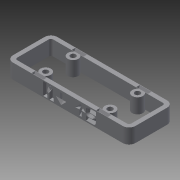
# Autodesk Inventor part: dualBaccable-ucan_fysect_middle
Saved by Autodesk Inventor 2014 SP2 (Build 180246200, 246)
## iProperties
Created: 2025-01-14
Part Number: dualBaccable-ucan_fysect_middle
Material: Generic
Document SubType Name: Sheet Metal
Designer: GauchoHP
Density: 1 g/cm^3
Sheet Metal Rule: Default_mm
Appearance: Default
Author: GauchoHP
Autodesk Inventor part; units mm, degrees
ref_plane "YZ Plane" through (0, 0, 0) normal (1, 0, 0) x (0, 1, 0)
ref_plane "XZ Plane" through (0, 0, 0) normal (0, 1, 0) x (-1, 0, 0)
ref_plane "XY Plane" through (0, 0, 0) normal (0, 0, 1) x (1, 0, 0)
sketch "Sketch1" plane through (0, 0, 0) normal (0, 0, 1) x (1, 0, 0)
  line L0 (-8.892067, 9.824871) -> (43.107933, 9.824871)
  line L1 (46.107933, 6.824871) -> (46.107933, -8.175129)
  line L2 (43.107933, -11.175129) -> (-8.892067, -11.175129)
  line L3 (-11.892067, -8.175129) -> (-11.892067, 6.824871)
  arc A0 (-8.892067, 9.824871) -> (-11.892067, 6.824871) centre (-8.892067, 6.824871) ccw
  arc A1 (46.107933, 6.824871) -> (43.107933, 9.824871) centre (43.107933, 6.824871) ccw
  arc A2 (43.107933, -11.175129) -> (46.107933, -8.175129) centre (43.107933, -8.175129) ccw
  arc A3 (-11.892067, -8.175129) -> (-8.892067, -11.175129) centre (-8.892067, -8.175129) ccw
  line L4 (43.107933, 7.824871) -> (-8.892067, 7.824871)
  arc A4 (-8.892067, 7.824871) -> (-9.892067, 6.824871) centre (-8.892067, 6.824871) ccw
  line L5 (-9.892067, 6.824871) -> (-9.892067, -8.175129)
  arc A5 (-9.892067, -8.175129) -> (-8.892067, -9.175129) centre (-8.892067, -8.175129) ccw
  line L6 (-8.892067, -9.175129) -> (43.107933, -9.175129)
  arc A6 (43.107933, -9.175129) -> (44.107933, -8.175129) centre (43.107933, -8.175129) ccw
  line L7 (44.107933, -8.175129) -> (44.107933, 6.824871)
  arc A7 (44.107933, 6.824871) -> (43.107933, 7.824871) centre (43.107933, 6.824871) ccw
  circle A8 centre (2.607933, -7.175129) radius 2.5
  circle A9 centre (2.607933, -7.175129) radius 1.25
  circle A10 centre (2.607933, 5.824871) radius 2.5
  circle A11 centre (2.607933, 5.824871) radius 1.25
  circle A12 centre (33.107933, 5.824871) radius 2.5
  circle A13 centre (33.107933, 5.824871) radius 1.25
  circle A14 centre (33.107933, -7.175129) radius 2.5
  circle A15 centre (33.107933, -7.175129) radius 1.25
  point P0 (0, 0)
  point P1 (-11.892067, 9.824871)
  point P2 (46.107933, 9.824871)
  point P3 (-11.892067, -11.175129)
  dimension "d0" = 58
  dimension "d1" = 21
  dimension "d2" = 3
  dimension "d5" = 2
  dimension "d6" = 5
  dimension "d7" = 2.5
  dimension "d8" = 5
  dimension "d9" = 2.5
  dimension "d10" = 5
  dimension "d11" = 2.5
  dimension "d12" = 5
  dimension "d13" = 2.5
  dimension "d14" = 30.5
  dimension "d15" = 30.5
  dimension "d16" = 13
  dimension "d17" = 2
  dimension "d18" = 11
  dimension "d19" = 11
  constraints: 16 centre point, 16 end point, 16 point on circle, 8 tangent, 6 point on line, 4 coincident, 4 parallel, 3 equal radius, 2 perpendicular, 1 horizontal, 7 other
  measures "d0" distance of point (-11.892, 9.825) point (46.108, 9.825)
  measures "d1" distance of point (-11.892, -11.175) point (-11.892, 9.825)
  measures "d2" radius of A0
  measures "d5" distance between parallel lines of L4 L0
  measures "d6" diameter of A8
  measures "d7" diameter of A9
  measures "d8" diameter of A10
  measures "d9" diameter of A11
  measures "d10" diameter of A12
  measures "d11" diameter of A13
  measures "d12" diameter of A14
  measures "d13" diameter of A15
  measures "d14" distance of A12.centre A10.centre
  measures "d15" distance of A14.centre A8.centre
  measures "d16" distance of A8.centre A10.centre
  measures "d17" distance from line of L6 A8.centre
  measures "d18" distance from line of L7 A12.centre
  measures "d19" distance from line of L7 A14.centre
extrude "Extrusion1" add sketch "Sketch1" along normal blind 7 contours L0 A1 L1 A2 L2 A3 L3 A0 | A12 L4 | L4 A12 | A10 L4 | L4 A10 | A14 L6 | L6 A14 | A8 L6 | L6 A8
sketch "Sketch2" plane through (0, 0, 7) normal (0, 0, 1) x (1, 0, 0)
  circle A0 centre (2.607933, 5.824871) radius 1.25
  line L0 (43.107933, 9.824871) -> (-8.892067, 9.824871)
  line L1 (-8.892067, -11.175129) -> (43.107933, -11.175129)
  circle A1 centre (33.107933, -7.175129) radius 1.25
  circle A2 centre (33.107933, 5.824871) radius 1.25
  circle A3 centre (2.607933, -7.175129) radius 1.25
  line L2 (-0.142067, 9.174871) -> (5.357933, 9.174871)
  line L3 (5.357933, 9.174871) -> (5.357933, 8.474871)
  line L4 (5.357933, 8.474871) -> (-0.142067, 8.474871)
  line L5 (-0.142067, 8.474871) -> (-0.142067, 9.174871)
  line L6 (35.857933, 9.174871) -> (30.357933, 9.174871)
  line L7 (30.357933, 9.174871) -> (30.357933, 8.474871)
  line L8 (30.357933, 8.474871) -> (35.857933, 8.474871)
  line L9 (35.857933, 8.474871) -> (35.857933, 9.174871)
  line L10 (30.357933, -9.825129) -> (35.857933, -9.825129)
  line L11 (35.857933, -9.825129) -> (35.857933, -10.525129)
  line L12 (35.857933, -10.525129) -> (30.357933, -10.525129)
  line L13 (30.357933, -10.525129) -> (30.357933, -9.825129)
  line L14 (-0.142067, -9.825129) -> (5.357933, -9.825129)
  line L15 (5.357933, -9.825129) -> (5.357933, -10.525129)
  line L16 (5.357933, -10.525129) -> (-0.142067, -10.525129)
  line L17 (-0.142067, -10.525129) -> (-0.142067, -9.825129)
  point P0 (0, 0)
  dimension "d20" = 5.5
  dimension "d21" = 0.7
  dimension "d22" = 0.65
  dimension "d23" = 2.75
  dimension "d24" = 0.7
  dimension "d25" = 0.65
  dimension "d27" = 5.5
  dimension "d29" = 2.75
  dimension "d30" = 5.5
  dimension "d31" = 0.7
  dimension "d32" = 0.65
  dimension "d33" = 2.75
  dimension "d34" = 0.7
  dimension "d35" = 5.5
  dimension "d36" = 2.75
  dimension "d37" = 0.65
  constraints: 32 end point, 8 parallel, 4 horizontal, 4 perpendicular
  measures "d20" distance of L2.start L2.end
  measures "d21" distance of L2.end L3.end
  measures "d22" distance between parallel lines of L0 L2
  measures "d23" distance from line of L3 A0.centre
  measures "d24" distance of L6.end L7.end
  measures "d25" distance between parallel lines of L0 L6
  measures "d27" distance of L6.start L6.end
  measures "d29" distance from line of L7 A2.centre
  measures "d30" distance of L10.start L10.end
  measures "d31" distance of L10.end L11.end
  measures "d32" distance between parallel lines of L1 L12
  measures "d33" distance from line of L13 A1.centre
  measures "d34" distance of L14.end L15.end
  measures "d35" distance of L14.start L14.end
  measures "d36" distance from line of L17 A3.centre
  measures "d37" distance between parallel lines of L1 L16
extrude "Extrusion2" cut sketch "Sketch2" against normal blind 1.2 contours L2 L3 L4 L5 | L9 L8 L7 L6 | L10 L11 L12 L13 | L14 L15 L16 L17
chamfer "Chamfer1" distance 0.5 distance2 1.2 1 edges at (2.6079, -9.8251, 7) measured on face at (2.6079, -9.3251, 7)
chamfer "Chamfer2" distance 0.5 distance2 1.2 1 edges at (2.6079, -10.5251, 7) measured on face at (2.6079, -10.6251, 7)
chamfer "Chamfer3" distance 0.5 distance2 1.2 1 edges at (33.1079, -9.8251, 7) measured on face at (33.1079, -9.3251, 7)
chamfer "Chamfer4" distance 0.5 distance2 1.2 1 edges at (33.1079, -10.5251, 7) measured on face at (33.1079, -10.6251, 7)
chamfer "Chamfer5" distance 0.5 distance2 1.2 1 edges at (33.1079, 8.4749, 7) measured on face at (33.1079, 7.9749, 7)
chamfer "Chamfer6" distance 0.5 distance2 1.2 1 edges at (33.1079, 9.1749, 7) measured on face at (33.1079, 9.6749, 7)
chamfer "Chamfer7" distance 0.5 distance2 1.2 1 edges at (2.6079, 8.4749, 7) measured on face at (2.6079, 7.9749, 7)
chamfer "Chamfer8" distance 0.5 distance2 1.2 1 edges at (2.6079, 9.1749, 7) measured on face at (2.6079, 9.6749, 7)
sketch "Sketch3" plane through (0, 0, 0) normal (0, 0, -1) x (-1, 0, 0)
  circle A0 centre (-2.607933, -7.175129) radius 1.25
  line L0 (-43.107933, -11.175129) -> (8.892067, -11.175129)
  line L1 (8.892067, 9.824871) -> (-43.107933, 9.824871)
  circle A1 centre (-33.107933, 5.824871) radius 1.25
  circle A2 centre (-33.107933, -7.175129) radius 1.25
  circle A3 centre (-2.607933, 5.824871) radius 1.25
  line L2 (0.142067, -10.525129) -> (-5.357933, -10.525129)
  line L3 (-5.357933, -10.525129) -> (-5.357933, -9.825129)
  line L4 (-5.357933, -9.825129) -> (0.142067, -9.825129)
  line L5 (0.142067, -9.825129) -> (0.142067, -10.525129)
  line L6 (-35.857933, -10.525129) -> (-30.357933, -10.525129)
  line L7 (-30.357933, -10.525129) -> (-30.357933, -9.825129)
  line L8 (-30.357933, -9.825129) -> (-35.857933, -9.825129)
  line L9 (-35.857933, -9.825129) -> (-35.857933, -10.525129)
  line L10 (-30.357933, 8.474871) -> (-35.857933, 8.474871)
  line L11 (-35.857933, 8.474871) -> (-35.857933, 9.174871)
  line L12 (-35.857933, 9.174871) -> (-30.357933, 9.174871)
  line L13 (-30.357933, 9.174871) -> (-30.357933, 8.474871)
  line L14 (0.142067, 8.474871) -> (-5.357933, 8.474871)
  line L15 (-5.357933, 8.474871) -> (-5.357933, 9.174871)
  line L16 (-5.357933, 9.174871) -> (0.142067, 9.174871)
  line L17 (0.142067, 9.174871) -> (0.142067, 8.474871)
  point P0 (0, 0)
  point P1 (0, -1.350259)
  dimension "d64" = 5.5
  dimension "d65" = 0.7
  dimension "d66" = 0.65
  dimension "d67" = 2.75
  dimension "d68" = 0.7
  dimension "d69" = 0.65
  dimension "d70" = 5.5
  dimension "d71" = 2.75
  dimension "d72" = 5.5
  dimension "d73" = 0.7
  dimension "d74" = 0.65
  dimension "d75" = 2.75
  dimension "d76" = 0.7
  dimension "d77" = 5.5
  dimension "d78" = 2.75
  dimension "d79" = 0.65
  constraints: 36 end point, 8 parallel, 4 centre point, 4 perpendicular
  measures "d64" distance of L2.start L2.end
  measures "d65" distance of L2.end L3.end
  measures "d66" distance between parallel lines of L0 L2
  measures "d67" distance from line of L3 A0.centre
  measures "d68" distance of L6.end L7.end
  measures "d69" distance between parallel lines of L0 L6
  measures "d70" distance of L6.start L6.end
  measures "d71" distance from line of L7 A2.centre
  measures "d72" distance of L10.start L10.end
  measures "d73" distance of L10.end L11.end
  measures "d74" distance between parallel lines of L1 L12
  measures "d75" distance from line of L13 A1.centre
  measures "d76" distance of L14.end L15.end
  measures "d77" distance of L14.start L14.end
  measures "d78" distance from line of L17 A3.centre
  measures "d79" distance between parallel lines of L1 L16
extrude "Extrusion3" cut sketch "Sketch3" against normal blind 1.2 contours L2 L3 L4 L5 | L9 L8 L7 L6 | L10 L11 L12 L13 | L14 L15 L16 L17
chamfer "Chamfer9" distance 0.5 distance2 1.2 1 edges at (33.1079, 8.4749, 0) measured on face at (33.1079, 7.9749, 0)
chamfer "Chamfer10" distance 0.5 distance2 1.2 1 edges at (33.1079, 9.1749, 0) measured on face at (33.1079, 9.6749, 0)
chamfer "Chamfer11" distance 0.5 distance2 1.2 1 edges at (33.1079, -10.5251, 0) measured on face at (33.1079, -11.0251, 0)
chamfer "Chamfer12" distance 0.5 distance2 1.2 1 edges at (33.1079, -9.8251, 0) measured on face at (33.1079, -9.3251, 0)
chamfer "Chamfer13" distance 0.5 distance2 1.2 1 edges at (2.6079, 9.1749, 0) measured on face at (2.6079, 9.2749, 0)
chamfer "Chamfer14" distance 0.5 distance2 1.2 1 edges at (2.6079, 8.4749, 0) measured on face at (2.6079, 7.9749, 0)
chamfer "Chamfer15" distance 0.5 distance2 1.2 1 edges at (2.6079, -9.8251, 0) measured on face at (2.6079, -9.3251, 0)
chamfer "Chamfer16" distance 0.5 distance2 1.2 1 edges at (2.6079, -10.5251, 0) measured on face at (2.6079, -10.6251, 0)
sketch "Sketch4" plane through (-8.892067, -11.175129, 0) normal (0, -1, 0) x (1, 0, 0)
  line L0 (52, 0) -> (0, 0)
  line L1 (14.81046, 1) -> (15.81046, 1)
  line L2 (15.81046, 1) -> (15.81046, 4.585786)
  line L3 (15.81046, 6) -> (14.81046, 6)
  line L4 (14.81046, 6) -> (14.81046, 1)
  line L5 (17.81046, 6) -> (18.81046, 6)
  line L6 (18.81046, 6) -> (18.81046, 3)
  line L7 (18.81046, 1) -> (17.81046, 1)
  line L8 (17.81046, 1) -> (17.81046, 4.585786)
  line L9 (15.81046, 6) -> (16.81046, 5)
  line L10 (16.81046, 5) -> (17.81046, 6)
  line L11 (15.81046, 4.585786) -> (16.81046, 3.585786)
  line L12 (16.81046, 3.585786) -> (17.81046, 4.585786)
  line L13 (21.331649, 2.5) -> (22.831649, 1)
  line L14 (22.831649, 1) -> (24.331649, 2.5)
  line L15 (23.331649, 6) -> (22.331649, 6)
  line L16 (23.331649, 2.5) -> (23.331649, 6)
  line L17 (21.331649, 2.5) -> (22.331649, 2.5)
  line L18 (23.331649, 2.5) -> (24.331649, 2.5)
  line L19 (22.331649, 6) -> (22.331649, 2.5)
  line L20 (33.5, 4.5) -> (32, 6)
  line L21 (32, 6) -> (30.5, 4.5)
  line L22 (31.5, 1) -> (32.5, 1)
  line L23 (31.5, 4.5) -> (31.5, 1)
  line L24 (33.5, 4.5) -> (32.5, 4.5)
  line L25 (31.5, 4.5) -> (30.5, 4.5)
  line L26 (32.5, 1) -> (32.5, 4.5)
  line L27 (36.5, 4) -> (38, 4)
  line L28 (37.5, 3) -> (36, 3)
  line L29 (35, 2) -> (37.5, 2)
  line L30 (38, 1) -> (35, 1)
  line L31 (35, 1) -> (35, 2)
  line L32 (36, 6) -> (39, 6)
  line L33 (39, 6) -> (39, 5)
  line L34 (39, 5) -> (36.5, 5)
  line L35 (35, 4) -> (35, 5)
  line L36 (39, 2) -> (39, 3)
  line L37 (18.81046, 1) -> (18.81046, 3)
  arc A0 (36, 6) -> (35, 5) centre (36, 5) ccw
  arc A1 (39, 3) -> (38, 4) centre (38, 3) ccw
  arc A2 (38, 1) -> (39, 2) centre (38, 2) ccw
  arc A3 (35, 4) -> (36, 3) centre (36, 4) ccw
  arc A4 (36.5, 5) -> (36.5, 4) centre (36.5, 4.5) ccw
  arc A5 (37.5, 2) -> (37.5, 3) centre (37.5, 2.5) ccw
  point P0 (8.892067, 0)
  dimension "d106" = 1
  dimension "d107" = 3
  dimension "d108" = 5
  dimension "d109" = 1
  dimension "d110" = 1
  dimension "d111" = 1
  dimension "d112" = 1
  dimension "d116" = 5
  dimension "d118" = 1
  dimension "d121" = 1
  dimension "d122" = 5
  dimension "d123" = 5
  dimension "d125" = 4
  dimension "d134" = 1
  constraints: 74 end point, 12 point on circle, 11 perpendicular, 10 parallel, 8 tangent, 6 centre point, 5 horizontal, 3 equal radius
  measures "d106" distance of L7.end L7.start
  measures "d107" distance of L6.end L5.end
  measures "d108" distance of L1.end L3.start
  measures "d109" distance of L1.end L1.start
  measures "d110" distance between parallel lines of L9 L11
  measures "d111" distance between parallel lines of L12 L10
  measures "d112" distance of L15.end L15.start
  measures "d116" distance between parallel lines of L3 L1
  measures "d118" distance of L26.start L23.end
  measures "d121" distance between parallel lines of L0 L22
  measures "d122" distance from line of L15 L13.end
  measures "d123" distance from line of L22 L20.end
  measures "d125" distance between parallel lines of L6 L4
  measures "d134" distance between parallel lines of L0 L1
extrude "Extrusion4" cut sketch "Sketch4" against normal blind 1
chamfer "Chamfer18" distance 0.4 angle 45 16 edges at (28.6079, -11.1751, 6) (26.4008, -11.1751, 5.7071) (26.1079, -11.1751, 4.5) (26.4008, -11.1751, 3.2929) (27.8579, -11.1751, 3) (29.1079, -11.1751, 2.5) (27.3579, -11.1751, 2) (30.1079, -11.1751, 5.5) (28.8579, -11.1751, 5) (27.1079, -11.1751, 4.5) (28.3579, -11.1751, 4) (29.815, -11.1751, 3.7071) (30.1079, -11.1751, 2.5) (29.815, -11.1751, 1.2929) (27.6079, -11.1751, 1) (26.1079, -11.1751, 1.5)
chamfer "Chamfer19" distance 1 angle 45 4 edges at (22.1079, -11.1751, 4.5) (24.1079, -11.1751, 4.5) (12.9396, -11.1751, 2.5) (14.9396, -11.1751, 2.5)
chamfer "Chamfer22" distance 1 angle 45 10 edges at (23.1079, -10.1751, 1) (21.6079, -10.1752, 4.5) (22.3579, -10.1751, 5.25) (24.6079, -10.1752, 4.5) (23.8579, -10.1751, 5.25) (12.4396, -10.1752, 2.5) (13.1896, -10.1751, 1.75) (15.4396, -10.1752, 2.5) (14.6896, -10.1751, 1.75) (13.9396, -10.1751, 6)
chamfer "Chamfer23" distance 0.5 angle 45 15 edges at (28.6079, -10.1751, 6) (26.4008, -10.1751, 5.7071) (26.1079, -10.1751, 4.5) (26.4008, -10.1751, 3.2929) (27.8579, -10.1751, 3) (29.1079, -10.1751, 2.5) (27.3579, -10.1751, 2) (28.3579, -10.1751, 4) (29.815, -10.1751, 3.7071) (30.1079, -10.1751, 2.5) (29.815, -10.1751, 1.2929) (27.6079, -10.1751, 1) (27.2543, -10.1751, 4.1465) (27.2544, -10.1751, 4.8536) (28.8579, -10.1751, 5)
chamfer "Chamfer24" distance 0.5 angle 45 12 edges at (6.4184, -11.1751, 6) (7.4184, -11.1751, 5.5) (8.4184, -11.1751, 5.5) (9.4184, -11.1751, 6) (9.9184, -11.1751, 3.5) (5.9184, -11.1751, 3.5) (6.4184, -11.1751, 1) (9.4184, -11.1751, 1) (8.9184, -11.1751, 2.7929) (6.9184, -11.1751, 2.7929) (7.4184, -11.1751, 4.0858) (8.4184, -11.1751, 4.0858)
chamfer "Chamfer25" distance 0.5 angle 45 12 edges at (6.4184, -10.6751, 1) (6.9184, -10.6751, 2.7929) (9.9184, -10.6751, 3.5) (9.4184, -10.6751, 1) (5.9184, -10.6751, 3.5) (6.4184, -10.6751, 6) (7.4184, -10.6751, 5.5) (8.4184, -10.6751, 5.5) (9.4184, -10.6751, 6) (8.9184, -10.6751, 2.7929) (8.4184, -10.6751, 4.0858) (7.4184, -10.6751, 4.0858)
equation "\"BendRadius\" = Thickness"
equation "\"BendReliefWidth\" = Thickness"
equation "\"BendReliefDepth\" = 0.5 * Thickness"
equation "\"CornerReliefSize\" = 4 * Thickness"
equation "\"MinimumRemnant\" = 2 * Thickness"
equation "\"TransitionRadius\" = BendRadius"
equation "\"JacobiRadiusSize\" = BendRadius"
equation "\"GapSize\" = Thickness"
equation "\"Thickness\" = 0.5"
body "Solid1"
